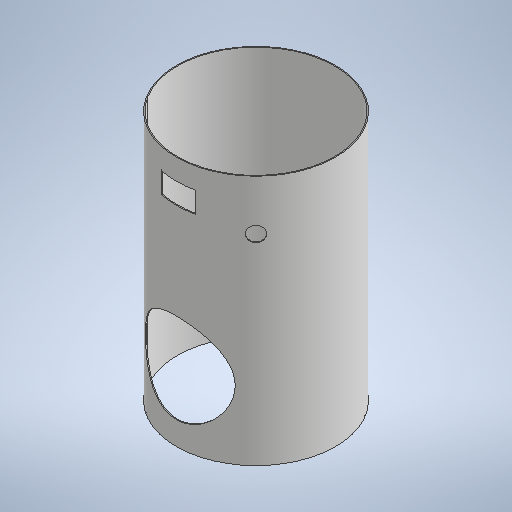
# Autodesk Inventor part: PRS 8110 main Shell_940
Saved by Autodesk Inventor 2026.2 (Build 302298000, 298)
## iProperties
Created: 2025-02-11
Part Number: PRS 8110 main Shell_940
Material: Steel
Document SubType Name: Sheet Metal
Designer: pokla
Mass: 197479 g
Surface Area: 84554.1 cm^2
Volume: 25156.5 cm^3
Density: 7.85 g/cm^3
Flat Pattern Width: 150 cm
Flat Pattern Length: 296.886 cm
Flat Pattern Area: 44532.9 cm^2
Sheet Metal Rule: Default_mm
Sheet Metal Width: 1500,000 mm
Sheet Metal Length: 2968,860 mm
Sheet Metal Area: 4453289,687 mm^2
Appearance: Default
Author: pokla
Autodesk Inventor part; units mm, degrees
sketch "Sketch13" plane through (0, 0, 0) normal (0, 0, 1) x (1, 0, 0)
  circle A0 centre (0, 0) radius 476 construction
  line L0 (0, 0) -> (0, -476)
  line L1 (0, 0) -> (-403.6709, -252.2416)
  line L2 (0, 0) -> (336.5828, -336.5828)
  line L3 (0, 0) -> (0, -476)
  line L4 (0, 0) -> (0, -476)
  line L5 (0, 0) -> (-424.1191, -216.0995)
  arc A1 (-403.6709, -252.2416) -> (0, -476) centre (0, 0) ccw
  dimension "d53" = 952
  dimension "d54" = 58
  dimension "d55" = 0
  dimension "d56" = 0
  dimension "d57" = 315
  dimension "d58" = 63
  constraints: 12 end point, 8 point on circle, 2 centre point, 2 coincident, 1 vertical
  measures "d53" diameter of A0
  measures "d54" angle of L0 L1
  measures "d55" distance between parallel lines of L0 L4
  measures "d56" distance between parallel lines of L0 L3
  measures "d58" angle of L0 L5
ref_plane "WeldJoint" through (0, 0, -10) normal (0.5299, -0.848, 0) x (0, 0, 1)
ref_plane "Outer" through (0, 0, -10) normal (0.454, -0.891, 0) x (0, 0, 1)
ref_plane "Clock_Feeder" through (0, 0, -10) normal (0.7071, 0.7071, 0) x (0, 0, 1)
ref_plane "Charging" through (0, 0, -10) normal (1, 0, 0) x (0, 0, 1)
ref_plane "Accsess" through (0, 0, -10) normal (1, 0, 0) x (0, 0, 1)
sketch "Sketch14" plane through (0, 0, -10) normal (0.5299, -0.848, 0) x (0, 0, 1)
  line L0 (1510, 470) -> (10, 470)
  line L1 (10, 470) -> (10, 476)
  line L2 (10, 476) -> (1510, 476)
  line L3 (1510, 476) -> (1510, 470)
  line L4 (10, 0) -> (825.0673, 0)
  point P0 (10, 473)
  dimension "d59" = 1500
  dimension "d60" = 6
  dimension "d61" = 952
  constraints: 10 end point, 2 horizontal, 2 parallel, 1 midpoint, 1 perpendicular, 1 vertical alignment
  measures "d59" distance of L1.end L2.end
  measures "d60" distance of L0.end L1.end
  measures "d61" diameter of L2 L4
revolve "Revolution2" add sketch "Sketch14" angle 359.9 about axis through (0, 0, 0) along (0, 0, 1)
sketch "Sketch AnglePlane_Feeder" plane through (0, 0, -10) normal (0.7071, 0.7071, 0) x (0, 0, 1)
  line L0 (10, -476) -> (10, 476) projected
  line L1 (10, 0) -> (1210, 0)
  line L2 (1210, 0) -> (1210, 476)
  line L3 (1210, 476) -> (10, 476)
  line L4 (10, 476) -> (10, 0)
  point P0 (10, -107.0767)
  point P1 (10, -107.886)
  dimension "d63" = 952
  dimension "d64" = 90
  dimension "frd_hght" = 1200
  constraints: 8 end point, 1 collinear, 1 horizontal, 1 parallel
  measures "d63" diameter of L3 L1
  measures "d64" angle of L2 L3
  measures "frd_hght" distance of L2.end L3.end
ref_plane "AnglePlane_Feeder" through (0, 0, 1200) normal (0.7071, -0.7071, 0) x (0.7071, 0.7071, 0)
sketch "Sketch16" plane through (0, 0, 1200) normal (0.7071, -0.7071, 0) x (0.7071, 0.7071, 0)
  circle A0 centre (0, 0) radius 45.5
  point P0 (0, -1200)
  point P1 (0, 0)
  point P2 (0, 0)
  point P3 (0, 0)
  dimension "d66" = 91
  constraints: 1 centre point, 1 coincident
  measures "d66" diameter of A0
extrude "Extrusion7" cut sketch "Sketch16" along normal through all
ref_plane "Work Plane16" through (0, 0, 0) normal (0, -1, 0) x (1, 0, 0)
sketch "Sketch17" plane through (0, 0, 0) normal (0, -1, 0) x (1, 0, 0)
  circle A0 centre (0, 408.5) radius 268.5
  line L0 (0, 140) -> (-495.5727, 140)
  point P0 (0, 0)
  dimension "d69" = 537
  dimension "d71" = 140
  constraints: 2 end point, 2 horizontal, 2 vertical alignment, 2 other
  measures "d71" distance from line of point (0, 0) L0
extrude "Extrusion8" cut sketch "Sketch17" along normal through all
sketch "Sketch19" plane through (0, 0, -10) normal (1, 0, 0) x (0, 0, 1)
  line L0 (10, 0) -> (1260, 0)
  line L1 (1260, 0) -> (1260, 476)
  line L2 (1260, 476) -> (10, 476)
  line L3 (10, 476) -> (10, 0)
  dimension "d74" = 1250
  dimension "d76" = 952
  dimension "d77" = 90
  constraints: 8 end point, 1 horizontal, 1 parallel, 1 perpendicular
  measures "d74" distance of L1.end L2.end
  measures "d76" diameter of L2 L0
  measures "d77" angle of L2 L1
ref_plane "Work Plane18" through (0, 0, 1250) normal (0, -1, 0) x (1, 0, 0)
sketch "Sketch20" plane through (0, 0, 1250) normal (0, -1, 0) x (1, 0, 0)
  line L0 (-103.5, 0) -> (103.5, 0)
  line L1 (103.5, 0) -> (103.5, 125)
  line L2 (103.5, 125) -> (-103.5, 125)
  line L3 (-103.5, 125) -> (-103.5, 0)
  point P0 (0, -1250)
  point P1 (0, 0)
  point P2 (0, 0)
  point P3 (0, 0)
  point P4 (0, 0)
  dimension "d78" = 207
  dimension "d79" = 125
  constraints: 8 end point, 2 parallel, 1 coincident, 1 horizontal, 1 midpoint, 1 perpendicular
  measures "d78" distance of L2.end L1.end
  measures "d79" distance of L1.end L0.end
extrude "Extrusion9" cut sketch "Sketch20" along normal through all
equation "\"BendRadius\" = Thickness"
equation "\"BendReliefWidth\" = Thickness"
equation "\"BendReliefDepth\" = 0.5 * Thickness"
equation "\"CornerReliefSize\" = 4 * Thickness"
equation "\"MinimumRemnant\" = 2 * Thickness"
equation "\"TransitionRadius\" = BendRadius"
equation "\"JacobiRadiusSize\" = BendRadius"
equation "\"GapSize\" = Thickness"
equation "\"Feeder_horisont_angle\" = 0"
equation "\"MAIN_filter_diam\" = 952"
equation "\"Hatch_Accsess_diameter\" = 535"
equation "\"Clock_Accsess_angle\" = 0"
equation "\"Clock_Charging_agnle\" = 0"
equation "\"Clock_Feeder_angle\" = 315deg"
equation "\"Clock_Outer_angle\" = 63deg"
equation "\"Clock_WeldJoint_angle\" = 58deg"
equation "\"Thickness\" = 6"
body "Solid2"
